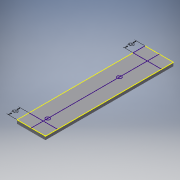
# Autodesk Inventor part: pickup plate 1
Saved by Autodesk Inventor 2017 (Build 210142000, 142)
## iProperties
Created: 2016-12-03
Part Number: pickup plate 1
Material: Generic
Document SubType Name: Modeling
Designer: Aditya
Density: 1 g/cm^3
Appearance: Default
Author: Aditya
Autodesk Inventor part; units mm, degrees
ref_plane "YZ Plane" through (0, 0, 0) normal (1, 0, 0) x (0, 1, 0)
ref_plane "XZ Plane" through (0, 0, 0) normal (0, 1, 0) x (-1, 0, 0)
ref_plane "XY Plane" through (0, 0, 0) normal (0, 0, 1) x (1, 0, 0)
sketch "Sketch1" plane through (0, 0, 0) normal (0, 1, 0) x (-1, 0, 0)
  line L0 (0, 0) -> (0, -114.3)
  line L1 (0, -114.3) -> (25.4, -114.3)
  line L2 (25.4, -114.3) -> (25.4, 0)
  line L3 (25.4, 0) -> (0, 0)
  dimension "d0" = 114.3
  dimension "d1" = 25.4
  constraints: 8 end point, 2 vertical, 1 horizontal, 1 perpendicular
  measures "d0" distance of L0.start L0.end
  measures "d1" distance of L0.end L1.end
extrude "Extrusion1" add sketch "Sketch1" along normal blind 3.175
sketch "Sketch2" plane through (0, 3.175, 0) normal (0, 1, 0) x (1, 0, 0)
  line L0 (-25.4, 0) -> (0, 0) projected
  line L1 (-25.4, 114.3) -> (-25.4, 0) projected
  line L2 (-25.4, 10.668) -> (0, 10.668)
  line L3 (0, 0) -> (0, 114.3) projected
  dimension "d4" = 10.668
  constraints: 2 end point, 2 point on line, 1 horizontal
  measures "d4" distance of L0.start L2.start
sketch "Sketch3" plane through (0, 3.175, 0) normal (0, 1, 0) x (1, 0, 0)
  line L0 (-25.4, 0) -> (0, 0) projected
  line L1 (-12.7, 0) -> (-12.7, 114.3)
  line L2 (0, 114.3) -> (-25.4, 114.3) projected
  constraints: 2 end point, 2 midpoint
sketch "Sketch4" plane through (0, 3.175, 0) normal (0, 1, 0) x (1, 0, 0)
  circle A0 centre (-12.7, 14.668) radius 1.85 projected
  circle A1 centre (-12.7, 78.668) radius 1.85 projected
  circle A2 centre (-12.7, 78.668) radius 1.85
  circle A3 centre (-12.7, 14.668) radius 1.85
  point P0 (0, 0)
  constraints: 2 centre point, 2 coincident, 2 concentric
sketch "Sketch5" plane through (0, 3.175, 0) normal (0, 1, 0) x (1, 0, 0)
  line L0 (0, 114.3) -> (-25.4, 114.3) projected
  line L1 (-25.4, 114.3) -> (-25.4, 103.632)
  line L2 (-25.4, 114.3) -> (-25.4, 0) projected
  line L3 (-25.4, 103.632) -> (0, 103.632)
  point P0 (0, 0)
  dimension "d5" = 10.668
  constraints: 4 end point, 1 perpendicular, 1 point on line
  measures "d5" distance of L0.end L1.end
body "Solid1"
